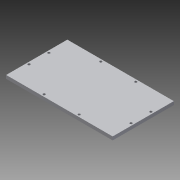
# Autodesk Inventor part: Base
Saved by Autodesk Inventor 2015 (Build 190159000, 159)
## iProperties
Created: 2015-05-15
Part Number: Base
Material: ABS Plastic
Document SubType Name: Modeling
Designer: carpenma
Density: 1.06 g/cm^3
Appearance: Smooth - White
Author: carpenma
Autodesk Inventor part; units mm, degrees
ref_plane "YZ Plane" through (0, 0, 0) normal (1, 0, 0) x (0, 1, 0)
ref_plane "XZ Plane" through (0, 0, 0) normal (0, 1, 0) x (-1, 0, 0)
ref_plane "XY Plane" through (0, 0, 0) normal (0, 0, 1) x (1, 0, 0)
sketch "Sketch1" plane through (0, 0, 0) normal (0, 1, 0) x (-1, 0, 0)
  line L0 (0, 0) -> (-298.45, 0)
  line L1 (-298.45, 0) -> (-298.45, 171.45)
  line L2 (-298.45, 171.45) -> (0, 171.45)
  line L3 (0, 171.45) -> (0, 0)
  dimension "d0" = 298.45
  dimension "d1" = 171.45
  constraints: 8 end point, 2 parallel, 1 horizontal, 1 perpendicular
  measures "d0" distance of L1.end L2.end
  measures "d1" distance of L0.end L1.end
extrude "Extrusion1" add sketch "Sketch1" along normal blind 9.525
sketch "Sketch3" plane through (0, 9.525, 0) normal (0, 1, 0) x (1, 0, 0)
  circle A0 centre (198.2183, -6.35) radius 3.3782 projected
  circle A1 centre (100.2317, -6.35) radius 3.3782 projected
  circle A2 centre (292.1, -57.8984) radius 3.3782 projected
  circle A3 centre (292.1, -113.5516) radius 3.3782 projected
  circle A4 centre (198.2183, -165.1) radius 3.3782 projected
  circle A5 centre (100.2317, -165.1) radius 3.3782 projected
  circle A6 centre (6.35, -57.8984) radius 3.3782 projected
  circle A7 centre (6.35, -113.5516) radius 3.3782 projected
  point P0 (0, 0)
extrude "Extrusion2" cut sketch "Sketch3" against normal up to next
fillet "Fillet1" radius 3.175 4 edges at (298.45, 4.7625, 171.45) (0, 4.7625, 171.45) (0, 4.7625, 0) (298.45, 4.7625, 0)
body "Solid1"
